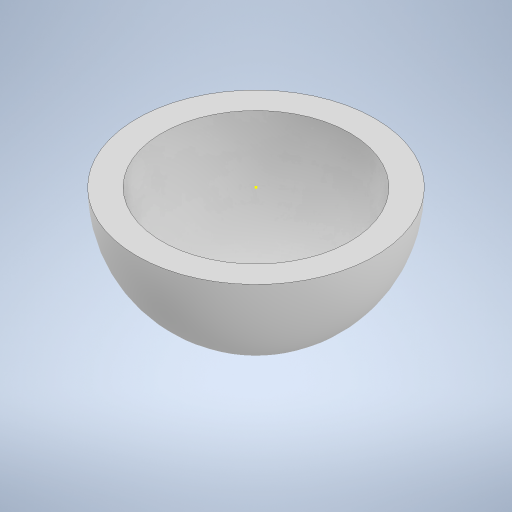
# Autodesk Inventor part: tail12.16
Saved by Autodesk Inventor 2023 (Build 270158000, 158)
## iProperties
Created: 2022-12-16
Part Number: tail12.16
Material: 一般
Document SubType Name: Modeling
Designer: ellie
Density: 1 g/cm^3
Appearance: 既定
Author: ellie
Autodesk Inventor part; units mm, degrees
ref_plane "YZ Plane" through (0, 0, 0) normal (1, 0, 0) x (0, 1, 0)
ref_plane "XZ Plane" through (0, 0, 0) normal (0, 1, 0) x (-1, 0, 0)
ref_plane "XY Plane" through (0, 0, 0) normal (0, 0, 1) x (1, 0, 0)
sketch "スケッチ1" plane through (0, 0, 0) normal (0, 1, 0) x (-1, 0, 0)
  circle A0 centre (0, 0) radius 37.5
  circle A1 centre (0, 0) radius 47.5
  line L0 (0, -47.5) -> (0, 47.5)
  point P0 (0, -37.5)
  point P1 (0, 37.5)
  dimension "d0" = 75
  dimension "d1" = 95
  dimension "d2" = 95
  constraints: 2 centre point, 2 coincident, 2 end point, 2 point on circle, 1 vertical
  measures "d0" diameter of A0
  measures "d1" diameter of A1
  measures "d2" distance of L0.start L0.end
sketch "スケッチ2" plane through (0, 0, 0) normal (0, 1, 0) x (-1, 0, 0)
  point P0 (0, 0)
revolve "回転1" add sketch "スケッチ1" angle 180 about axis through (0, 0, -47.5) along (0, 0, 1) picked at (43.8624, 3.0889) contours A0 L0 A1
